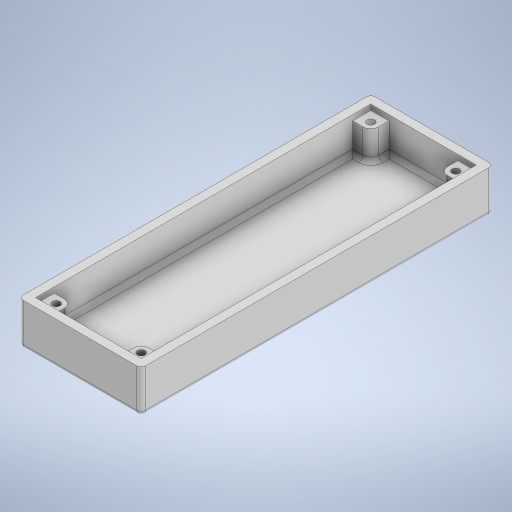
# Autodesk Inventor part: CaseBottom
Saved by Autodesk Inventor 2023 (Build 270158000, 158)
## iProperties
Created: 2022-10-21
Part Number: CaseBottom
Material: Generic
Document SubType Name: Modeling
Designer: Intern
Density: 1 g/cm^3
Appearance: Default
Author: Intern
Autodesk Inventor part; units mm, degrees
ref_plane "YZ Plane" through (0, 0, 0) normal (1, 0, 0) x (0, 1, 0)
ref_plane "XZ Plane" through (0, 0, 0) normal (0, 1, 0) x (-1, 0, 0)
ref_plane "XY Plane" through (0, 0, 0) normal (0, 0, 1) x (1, 0, 0)
sketch "Sketch1" plane through (0, 0, 0) normal (0, 1, 0) x (-1, 0, 0)
  line L0 (8.0502, -54.6054) -> (-23.4458, -54.6054)
  line L1 (-23.4458, -54.6054) -> (-23.4458, 45.4706)
  line L2 (-23.4458, 45.4706) -> (8.0502, 45.4706)
  line L3 (8.0502, 45.4706) -> (8.0502, -54.6054)
  line L4 (10.5902, -57.1454) -> (-25.9858, -57.1454)
  line L5 (-25.9858, -57.1454) -> (-25.9858, 48.0106)
  line L6 (-25.9858, 48.0106) -> (10.5902, 48.0106)
  line L7 (10.5902, 48.0106) -> (10.5902, -57.1454)
  point P0 (0, 0)
  point P1 (-7.6978, -57.1454)
  dimension "d0" = 100.076
  dimension "d1" = 31.496
  dimension "d2" = 2.54
  dimension "d3" = 2.54
  dimension "d4" = 2.54
  dimension "d5" = 2.54
  constraints: 16 end point, 4 parallel, 2 horizontal, 2 perpendicular, 1 midpoint
  measures "d0" distance of L0.end L1.end
  measures "d1" distance of L1.end L2.end
  measures "d2" distance between parallel lines of L3 L7
  measures "d3" distance between parallel lines of L1 L5
  measures "d4" distance from line of L0 point (-7.698, -57.145)
  measures "d5" distance between parallel lines of L6 L2
extrude "Extrusion1" add sketch "Sketch1" against normal blind 12.7508 contours L0 L1 L2 L3 | L4 L5 L6 L7
extrude "Extrusion2" cut sketch "Sketch1" against normal blind 10.2108 contours L0 L1 L2 L3
sketch "Sketch2" plane through (0, -10.2108, 0) normal (0, 1, 0) x (1, 0, 0)
  circle A0 centre (-5.0022, -42.4226) radius 1.143
  line L0 (-8.0502, -45.4706) -> (-8.0502, 54.6054) projected
  line L1 (23.4458, -45.4706) -> (-8.0502, -45.4706) projected
  arc A1 (-2.5892, -42.4226) -> (-5.0022, -40.0096) centre (-5.0022, -42.4226) ccw
  line L2 (-5.0022, -40.0096) -> (-8.0502, -40.0096)
  line L3 (-2.5892, -42.4226) -> (-2.5892, -45.4706)
  line L4 (23.4458, -45.4706) -> (-8.0502, -45.4706) projected
  line L5 (-8.0502, -45.4706) -> (-2.5892, -45.4706)
  line L6 (-8.0502, -40.0096) -> (-8.0502, -45.4706)
  line L7 (23.4458, 54.6054) -> (23.4458, -45.4706) projected
  line L8 (-8.0502, 54.6054) -> (23.4458, 54.6054) projected
  line L9 (-8.0502, 4.5674) -> (30.3732, 4.5674)
  line L10 (7.6978, -45.4706) -> (7.6978, 57.2864)
  circle A2 centre (20.3978, -42.4226) radius 1.143
  line L11 (23.4458, -45.4706) -> (23.4458, 54.6054)
  line L12 (-8.0502, -45.4706) -> (23.4458, -45.4706)
  arc A3 (20.3978, -40.0096) -> (17.9848, -42.4226) centre (20.3978, -42.4226) ccw
  line L13 (20.3978, -40.0096) -> (23.4458, -40.0096)
  line L14 (17.9848, -42.4226) -> (17.9848, -45.4706)
  line L15 (-8.0502, -45.4706) -> (23.4458, -45.4706)
  line L16 (23.4458, -40.0096) -> (23.4458, -45.4706)
  circle A4 centre (-5.0022, 51.5574) radius 1.143
  line L17 (23.4458, 54.6054) -> (-8.0502, 54.6054)
  arc A5 (-5.0022, 49.1444) -> (-2.5892, 51.5574) centre (-5.0022, 51.5574) ccw
  line L18 (-5.0022, 49.1444) -> (-8.0502, 49.1444)
  line L19 (-2.5892, 51.5574) -> (-2.5892, 54.6054)
  line L20 (23.4458, 54.6054) -> (-8.0502, 54.6054)
  line L21 (-8.0502, 54.6054) -> (-2.5892, 54.6054)
  line L22 (-8.0502, 49.1444) -> (-8.0502, 54.6054)
  circle A6 centre (20.3978, 51.5574) radius 1.143
  arc A7 (17.9848, 51.5574) -> (20.3978, 49.1444) centre (20.3978, 51.5574) ccw
  line L23 (17.9848, 51.5574) -> (17.9848, 54.6054)
  line L24 (-8.0502, 54.6054) -> (23.4458, 54.6054)
  line L25 (20.3978, 49.1444) -> (23.4458, 49.1444)
  line L26 (-8.0502, 54.6054) -> (23.4458, 54.6054)
  line L27 (23.4458, 49.1444) -> (23.4458, 54.6054)
  point P0 (0, 0)
  point P1 (7.6978, 54.6054)
  dimension "d10" = 2.286
  dimension "d11" = 3.048
  dimension "d12" = 3.048
  dimension "d13" = 4.826
  constraints: 46 end point, 25 symmetric about line, 8 centre point, 8 point on circle, 6 point on line, 4 coincident, 2 collinear, 2 midpoint, 2 perpendicular, 1 horizontal, 1 vertical, 6 other
  measures "d10" diameter of A0
  measures "d11" distance from line of L0 A0.centre
  measures "d12" distance from line of L1 A0.centre
  measures "d13" diameter of A1
extrude "Extrusion3" add sketch "Sketch2" along normal blind 8.636 contours L0 L2 A1 L3 L1 | L0 L8 L19 A5 L18 | L14 A3 L13 L7 L1 | L25 A7 L23 L8 L7
fillet "Fillet1" radius 1.27 8 edges at (7.6978, -12.7508, 48.0106) (25.9858, -6.3754, 48.0106) (25.9858, -12.7508, -4.5674) (25.9858, -6.3754, -57.1454) (-10.5902, -6.3754, 48.0106) (-10.5902, -12.7508, -4.5674) (-10.5902, -6.3754, -57.1454) (7.6978, -12.7508, -57.1454)
fillet "Fillet2" radius 1.27 16 edges at (-8.0502, -10.2108, -4.5674) (7.6978, -10.2108, -54.6054) (-6.5262, -10.2108, -49.1444) (-2.5892, -10.2108, -53.0814) (-3.296, -10.2108, -49.8511) (17.9848, -10.2108, -53.0814) (21.9218, -10.2108, -49.1444) (18.6915, -10.2108, -49.8511) (23.4458, -10.2108, -4.5674) (21.9218, -10.2108, 40.0096) (17.9848, -10.2108, 43.9466) (18.6915, -10.2108, 40.7164) (7.6978, -10.2108, 45.4706) (-2.5892, -10.2108, 43.9466) (-6.5262, -10.2108, 40.0096) (-3.296, -10.2108, 40.7164)
body "Solid1"
